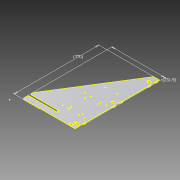
# Autodesk Inventor part: side_frame_v2
Saved by Autodesk Inventor 2013 (Build 170138000, 138)
## iProperties
Created: 2013-11-17
Part Number: side_frame_v2
Material: Generic
Document SubType Name: Modeling
Designer: Masta
Density: 1 g/cm^3
Author: Masta
Autodesk Inventor part; units mm, degrees
ref_plane "YZ Plane" through (0, 0, 0) normal (1, 0, 0) x (0, 1, 0)
ref_plane "XZ Plane" through (0, 0, 0) normal (0, 1, 0) x (-1, 0, 0)
ref_plane "XY Plane" through (0, 0, 0) normal (0, 0, 1) x (1, 0, 0)
sketch "Sketch1" plane through (0, 0, 0) normal (0, 0, 1) x (1, 0, 0)
  line L0 (255.7808, 350.0828) -> (255.7808, 358.8828)
  line L1 (251.6808, 67.29) -> (255.7808, 67.29)
  line L2 (255.7808, 67.29) -> (255.7808, 76.09)
  line L3 (255.7808, 76.09) -> (251.6808, 76.09)
  line L4 (251.6808, 76.09) -> (251.6808, 194.9901)
  line L5 (251.6808, 32.5401) -> (100.8808, 32.5401)
  line L6 (231.7439, 44.5401) -> (223.7479, 44.5401)
  line L7 (230.5808, 213.3401) -> (234.5808, 213.3401)
  line L8 (234.5808, 211.5401) -> (239.6808, 211.5401)
  line L9 (251.6808, 57.7345) -> (239.6808, 57.7345)
  line L10 (239.6808, 57.7345) -> (239.6808, 59.5345)
  line L11 (230.5808, 53.3345) -> (234.5808, 53.3345)
  line L12 (234.5808, 51.5345) -> (239.6808, 51.5345)
  line L13 (239.6808, 59.5345) -> (234.5808, 59.5345)
  line L14 (234.5808, 53.3345) -> (234.5808, 51.5345)
  line L15 (239.6808, 53.3345) -> (251.6808, 53.3345)
  line L16 (239.6808, 51.5345) -> (239.6808, 53.3345)
  line L17 (251.6808, 57.7345) -> (251.6808, 67.29)
  line L18 (251.6808, 217.7401) -> (239.6808, 217.7401)
  line L19 (255.7808, 236.0901) -> (251.6808, 236.0901)
  line L20 (251.6808, 236.0901) -> (251.6808, 350.0828)
  line L21 (255.7808, 203.7901) -> (251.6808, 203.7901)
  line L22 (251.6808, 194.9901) -> (255.7808, 194.9901)
  line L23 (255.7808, 194.9901) -> (255.7808, 203.7901)
  line L24 (251.6808, 227.2901) -> (251.6808, 217.7401)
  line L25 (251.6808, 213.3401) -> (251.6808, 203.7901)
  line L26 (251.6808, 382.3828) -> (255.7808, 382.3828)
  line L27 (255.7808, 382.3828) -> (255.7808, 391.1828)
  line L28 (255.7808, 391.1828) -> (251.6808, 391.1828)
  line L29 (251.6808, 391.1828) -> (251.6808, 400.5401)
  line L30 (255.7808, 358.8828) -> (251.6808, 358.8828)
  line L31 (251.6808, 350.0828) -> (255.7808, 350.0828)
  line L32 (73.8808, 35.5401) -> (73.8808, 51.1401)
  line L33 (239.6808, 211.5401) -> (239.6808, 213.3401)
  line L34 (230.5808, 217.7401) -> (230.5808, 213.3401)
  line L35 (73.8808, 77.5401) -> (226.2808, 400.5401)
  line L36 (234.5808, 217.7401) -> (230.5808, 217.7401)
  line L37 (234.5808, 217.7401) -> (234.5808, 219.5401)
  line L38 (251.6808, 400.5401) -> (226.2808, 400.5401)
  line L39 (239.6808, 213.3401) -> (251.6808, 213.3401)
  line L40 (231.7439, 36.5395) -> (223.7482, 36.5395)
  line L41 (239.6808, 219.5401) -> (234.5808, 219.5401)
  line L42 (98.8808, 30.5401) -> (78.8808, 30.5401)
  line L43 (234.5808, 213.3401) -> (234.5808, 211.5401)
  line L44 (230.5808, 372.825) -> (230.5808, 368.425)
  line L45 (234.5808, 372.825) -> (230.5808, 372.825)
  line L46 (234.5808, 372.825) -> (234.5808, 374.625)
  line L47 (251.6808, 372.825) -> (239.6808, 372.825)
  line L48 (230.5808, 368.425) -> (234.5808, 368.425)
  line L49 (239.6808, 368.425) -> (251.6808, 368.425)
  line L50 (234.5808, 366.625) -> (239.6808, 366.625)
  line L51 (239.6808, 374.625) -> (234.5808, 374.625)
  line L52 (234.5808, 368.425) -> (234.5808, 366.625)
  line L53 (251.6808, 372.825) -> (251.6808, 382.3828)
  line L54 (251.6808, 368.425) -> (251.6808, 358.8828)
  line L55 (230.5808, 57.7345) -> (230.5808, 53.3345)
  line L56 (234.5808, 57.7345) -> (230.5808, 57.7345)
  line L57 (234.5808, 57.7345) -> (234.5808, 59.5345)
  line L58 (239.6808, 366.625) -> (239.6808, 368.425)
  line L59 (239.6808, 372.825) -> (239.6808, 374.625)
  line L60 (78.8808, 56.1401) -> (148.8808, 56.1401)
  line L61 (78.8808, 56.1401) -> (73.8808, 51.1401)
  line L62 (78.8808, 64.9401) -> (148.8808, 64.9401)
  line L63 (73.8808, 69.9401) -> (73.8808, 77.5401)
  line L64 (78.8808, 64.9401) -> (73.8808, 69.9401)
  line L65 (251.6808, 227.2901) -> (255.7808, 227.2901)
  line L66 (255.7808, 227.2901) -> (255.7808, 236.0901)
  line L67 (239.6808, 217.7401) -> (239.6808, 219.5401)
  line L68 (78.8808, 30.5401) -> (73.8808, 35.5401)
  line L69 (100.8808, 32.5401) -> (98.8808, 30.5401)
  line L70 (251.6808, 32.5401) -> (251.6808, 53.3345)
  line L71 (136.6808, 189.5401) -> (231.6808, 189.5401) construction
  line L72 (231.6808, 189.5401) -> (231.6808, 93.5401) construction
  line L73 (231.6808, 93.5401) -> (136.6808, 93.5401) construction
  line L74 (136.6808, 93.5401) -> (136.6808, 189.5401) construction
  line L75 (164.6808, 93.5401) -> (208.6808, 93.5401) construction
  line L76 (208.6808, 93.5401) -> (208.6808, 187.5401) construction
  line L77 (208.6808, 187.5401) -> (164.6808, 187.5401) construction
  line L78 (164.6808, 187.5401) -> (164.6808, 93.5401) construction
  line L79 (160.3808, 93.5401) -> (208.6808, 93.5401) construction
  line L80 (208.6808, 93.5401) -> (208.6808, 168.5401) construction
  line L81 (208.6808, 168.5401) -> (160.3808, 168.5401) construction
  line L82 (160.3808, 168.5401) -> (160.3808, 93.5401) construction
  line L83 (208.6808, 168.5401) -> (208.6808, 174.8401) construction
  arc A0 (148.8808, 56.1401) -> (148.8808, 64.9401) centre (148.8808, 60.5401) ccw
  arc A1 (231.7439, 36.5395) -> (231.7439, 44.5401) centre (231.7439, 40.5398) ccw
  arc A2 (223.7479, 44.5401) -> (223.7482, 36.5395) centre (223.7482, 40.5398) ccw
  point P0 (0, 0)
  point P1 (219.7479, 40.5401)
  dimension "d0" = 177.8
  dimension "d9" = 95
  dimension "d10" = 96
  dimension "d11" = 44
  dimension "d12" = 94
  dimension "d15" = 48.3
  dimension "d16" = 75
  dimension "d18" = 6.3
  dimension "d19" = 23
  dimension "d20" = 20
  dimension "d21" = 63
  dimension "d22" = 4.1
  dimension "d23" = 8.8
  constraints: 168 end point, 17 collinear, 11 coincident, 7 parallel, 7 point on circle, 5 tangent, 4 horizontal, 3 centre point, 3 perpendicular, 1 vertical
  measures "d0" distance between parallel lines of L32 L70
  measures "d9" distance of L72.end L73.end
  measures "d10" distance of L71.end L72.end
  measures "d11" distance of L77.end L76.end
  measures "d12" distance of L75.end L76.end
  measures "d15" distance of L81.end L80.end
  measures "d16" distance of L80.end L75.end
  measures "d18" distance of L80.end L83.end
  measures "d19" distance between parallel lines of L72 L80
  measures "d20" distance between parallel lines of L4 L72
  measures "d21" distance between parallel lines of L42 L73
  measures "d22" distance between parallel lines of L2 L17
  measures "d23" distance of L1.end L2.end
extrude "Extrusion1" add sketch "Sketch1" against normal blind 4
hole "Hole1" at (136.6808, 189.5401, 0) at (136.6808, 93.5401, 0) at (231.6808, 93.5401, 0) at (231.6808, 189.5401, 0) at (160.3808, 93.5401, 0) at (208.6808, 93.5401, 0) at (208.6808, 174.8401, 0) at (160.3808, 168.5401, 0) at (164.6808, 93.5401, 0) at (164.6808, 187.5401, 0) at (208.6808, 187.5401, 0) direction (0, 0, -1) diameter 3.6 end through all
sketch "Sketch2" plane through (0, 0, 0) normal (0, 0, 1) x (1, 0, 0)
  line L0 (78.8808, 64.9401) -> (148.8808, 64.9401) projected
  line L1 (251.6808, 76.09) -> (251.6808, 194.9901) projected
  line L2 (162.1808, 104.9401) -> (212.1808, 104.9401) construction
  line L3 (212.1808, 104.9401) -> (212.1808, 254.9401) construction
  line L4 (212.1808, 254.9401) -> (162.1808, 254.9401) construction
  line L5 (162.1808, 254.9401) -> (162.1808, 104.9401) construction
  line L6 (162.1808, 104.9401) -> (212.1808, 254.9401) construction
  line L7 (212.1808, 104.9401) -> (162.1808, 254.9401) construction
  line L8 (129.6808, 69.9401) -> (244.6808, 69.9401) construction
  line L9 (244.6808, 69.9401) -> (244.6808, 289.9401) construction
  line L10 (244.6808, 289.9401) -> (129.6808, 289.9401) construction
  line L11 (129.6808, 289.9401) -> (129.6808, 69.9401) construction
  line L12 (129.6808, 69.9401) -> (244.6808, 289.9401) construction
  line L13 (244.6808, 69.9401) -> (129.6808, 289.9401) construction
  point P0 (0, 0)
  point P1 (187.1808, 179.9401)
  point P2 (187.1808, 179.9401)
  dimension "d33" = 50
  dimension "d34" = 150
  dimension "d35" = 115
  dimension "d36" = 220
  dimension "d37" = 5
  dimension "d38" = 7
  constraints: 24 end point, 5 midpoint, 4 coincident, 4 parallel, 2 horizontal, 2 perpendicular
  measures "d33" distance of L4.end L3.end
  measures "d34" distance of L3.end L2.end
  measures "d35" distance of L10.end L9.end
  measures "d36" distance of L9.end L8.end
  measures "d37" distance between parallel lines of L8 L0
  measures "d38" distance between parallel lines of L1 L9
hole "Hole2" at (162.1808, 254.9401, 0) at (162.1808, 104.9401, 0) at (212.1808, 104.9401, 0) at (212.1808, 254.9401, 0) direction (0, 0, -1) diameter 4.6 end through all
sketch "Sketch3" plane through (0, 0, 0) normal (0, 0, 1) x (1, 0, 0)
  line L0 (226.2808, 400.5401) -> (73.8808, 77.5401) projected
  line L1 (73.8808, 77.5401) -> (73.8808, 69.9401) projected
  line L2 (73.8808, 69.9401) -> (78.8808, 64.9401) projected
  line L3 (78.8808, 56.1401) -> (73.8808, 51.1401) projected
  line L4 (73.8808, 51.1401) -> (73.8808, 35.5401) projected
  line L5 (73.8808, 35.5401) -> (78.8808, 30.5401) projected
  line L6 (98.8808, 30.5401) -> (100.8808, 32.5401) projected
  line L7 (234.5808, 374.625) -> (239.6808, 374.625) projected
  line L8 (78.8808, 64.9401) -> (28.8808, 64.9401)
  line L9 (28.8808, 64.9401) -> (23.8808, 69.9401)
  line L10 (23.8808, 77.5401) -> (23.8808, 69.9401)
  line L11 (23.8808, 77.5401) -> (226.2808, 400.5401)
  line L12 (78.8808, 56.1401) -> (28.8808, 56.1401)
  line L13 (28.8808, 56.1401) -> (23.8808, 51.1401)
  line L14 (23.8808, 51.1401) -> (23.8808, 35.5401)
  line L15 (78.8808, 30.5401) -> (28.8808, 30.5401)
  line L16 (23.8808, 35.5401) -> (28.8808, 30.5401)
  point P0 (0, 0)
  point P1 (230.5808, 53.3345)
  point P2 (234.5808, 51.5345)
  point P3 (239.6808, 51.5345)
  point P4 (239.6808, 59.5345)
  point P5 (234.5808, 59.5345)
  point P6 (230.5808, 57.7345)
  point P7 (251.6808, 67.29)
  point P8 (251.6808, 76.09)
  point P9 (251.6808, 194.9901)
  point P10 (251.6808, 203.7901)
  point P11 (239.6808, 211.5401)
  point P12 (234.5808, 211.5401)
  point P13 (230.5808, 213.3401)
  point P14 (230.5808, 217.7401)
  point P15 (234.5808, 219.5401)
  point P16 (239.6808, 219.5401)
  point P17 (251.6808, 227.2901)
  point P18 (251.6808, 236.0901)
  point P19 (251.6808, 350.0828)
  point P20 (251.6808, 358.8828)
  point P21 (251.6808, 382.3828)
  point P22 (251.6808, 391.1828)
  point P23 (230.5808, 372.825)
  point P24 (230.5808, 368.425)
  point P25 (234.5808, 366.625)
  point P26 (239.6808, 366.625)
  dimension "d46" = 50
  dimension "d47" = 5
  dimension "d48" = 7.6
  constraints: 18 end point, 7 perpendicular, 2 coincident, 1 parallel
  measures "d46" distance of L2.end L8.end
  measures "d47" horizontal distance of L8.end L9.end
  measures "d48" distance of L10.start L9.end
extrude "Extrusion2" add sketch "Sketch3" against normal up to surface (4 mm away)
hole "Hole3" at (230.5808, 53.3345, 0) at (234.5808, 51.5345, 0) at (239.6808, 51.5345, 0) at (239.6808, 59.5345, 0) at (234.5808, 59.5345, 0) at (230.5808, 57.7345, 0) at (251.6808, 67.29, 0) at (251.6808, 76.09, 0) at (251.6808, 194.9901, 0) at (251.6808, 203.7901, 0) at (239.6808, 211.5401, 0) at (234.5808, 211.5401, 0) at (230.5808, 213.3401, 0) at (230.5808, 217.7401, 0) at (234.5808, 219.5401, 0) at (239.6808, 219.5401, 0) at (251.6808, 227.2901, 0) at (251.6808, 236.0901, 0) at (251.6808, 350.0828, 0) at (251.6808, 358.8828, 0) at (251.6808, 382.3828, 0) at (251.6808, 391.1828, 0) at (239.6808, 374.625, 0) at (234.5808, 374.625, 0) at (230.5808, 372.825, 0) at (230.5808, 368.425, 0) at (234.5808, 366.625, 0) at (239.6808, 366.625, 0) direction (0, 0, -1) diameter 1 end through all
sketch "Sketch4" plane through (0, 0, 0) normal (0, 0, 1) x (1, 0, 0)
  arc A0 (234.5808, 367.125) -> (235.0808, 366.625) centre (234.5808, 366.625) ccw projected
  line L0 (234.5808, 367.125) -> (234.5808, 368.425) projected
  line L1 (234.5808, 368.425) -> (231.0808, 368.425) projected
  arc A1 (230.5808, 368.925) -> (231.0808, 368.425) centre (230.5808, 368.425) ccw projected
  line L2 (230.5808, 368.925) -> (230.5808, 372.325) projected
  arc A2 (231.0808, 372.825) -> (230.5808, 372.325) centre (230.5808, 372.825) ccw projected
  line L3 (231.0808, 372.825) -> (234.5808, 372.825) projected
  line L4 (234.5808, 372.825) -> (234.5808, 374.125) projected
  arc A3 (235.0808, 374.625) -> (234.5808, 374.125) centre (234.5808, 374.625) ccw projected
  line L5 (235.0808, 374.625) -> (239.1808, 374.625) projected
  arc A4 (239.6808, 374.125) -> (239.1808, 374.625) centre (239.6808, 374.625) ccw projected
  line L6 (239.6808, 374.125) -> (239.6808, 372.825) projected
  line L7 (239.6808, 372.825) -> (251.6808, 372.825) projected
  line L8 (251.6808, 372.825) -> (251.6808, 381.8828) projected
  arc A5 (252.1808, 382.3828) -> (251.6808, 381.8828) centre (251.6808, 382.3828) ccw projected
  line L9 (252.1808, 382.3828) -> (255.7808, 382.3828) projected
  line L10 (255.7808, 382.3828) -> (255.7808, 391.1828) projected
  line L11 (255.7808, 391.1828) -> (252.1808, 391.1828) projected
  arc A6 (251.6808, 391.6828) -> (252.1808, 391.1828) centre (251.6808, 391.1828) ccw projected
  line L12 (251.6808, 391.6828) -> (251.6808, 400.5401) projected
  line L13 (251.6808, 400.5401) -> (226.2808, 400.5401) projected
  line L14 (226.2808, 400.5401) -> (23.8808, 77.5401) projected
  line L15 (23.8808, 77.5401) -> (23.8808, 69.9401) projected
  line L16 (23.8808, 69.9401) -> (28.8808, 64.9401) projected
  line L17 (28.8808, 64.9401) -> (148.8808, 64.9401) projected
  arc A7 (148.8808, 56.1401) -> (148.8808, 64.9401) centre (148.8808, 60.5401) ccw projected
  line L18 (148.8808, 56.1401) -> (28.8808, 56.1401) projected
  line L19 (28.8808, 56.1401) -> (23.8808, 51.1401) projected
  line L20 (23.8808, 51.1401) -> (23.8808, 35.5401) projected
  line L21 (23.8808, 35.5401) -> (28.8808, 30.5401) projected
  line L22 (28.8808, 30.5401) -> (98.8808, 30.5401) projected
  line L23 (98.8808, 30.5401) -> (100.8808, 32.5401) projected
  line L24 (100.8808, 32.5401) -> (251.6808, 32.5401) projected
  line L25 (251.6808, 32.5401) -> (251.6808, 53.3345) projected
  line L26 (251.6808, 53.3345) -> (239.6808, 53.3345) projected
  line L27 (239.6808, 53.3345) -> (239.6808, 52.0345) projected
  arc A8 (239.1808, 51.5345) -> (239.6808, 52.0345) centre (239.6808, 51.5345) ccw projected
  line L28 (239.1808, 51.5345) -> (235.0808, 51.5345) projected
  arc A9 (234.5808, 52.0345) -> (235.0808, 51.5345) centre (234.5808, 51.5345) ccw projected
  line L29 (234.5808, 52.0345) -> (234.5808, 53.3345) projected
  line L30 (234.5808, 53.3345) -> (231.0808, 53.3345) projected
  arc A10 (230.5808, 53.8345) -> (231.0808, 53.3345) centre (230.5808, 53.3345) ccw projected
  line L31 (230.5808, 53.8345) -> (230.5808, 57.2345) projected
  arc A11 (231.0808, 57.7345) -> (230.5808, 57.2345) centre (230.5808, 57.7345) ccw projected
  line L32 (231.0808, 57.7345) -> (234.5808, 57.7345) projected
  line L33 (234.5808, 57.7345) -> (234.5808, 59.0345) projected
  arc A12 (235.0808, 59.5345) -> (234.5808, 59.0345) centre (234.5808, 59.5345) ccw projected
  line L34 (235.0808, 59.5345) -> (239.1808, 59.5345) projected
  arc A13 (239.6808, 59.0345) -> (239.1808, 59.5345) centre (239.6808, 59.5345) ccw projected
  line L35 (239.6808, 59.0345) -> (239.6808, 57.7345) projected
  line L36 (239.6808, 57.7345) -> (251.6808, 57.7345) projected
  line L37 (251.6808, 57.7345) -> (251.6808, 66.79) projected
  arc A14 (252.1808, 67.29) -> (251.6808, 66.79) centre (251.6808, 67.29) ccw projected
  line L38 (252.1808, 67.29) -> (255.7808, 67.29) projected
  line L39 (255.7808, 67.29) -> (255.7808, 76.09) projected
  line L40 (255.7808, 76.09) -> (252.1808, 76.09) projected
  arc A15 (251.6808, 76.59) -> (252.1808, 76.09) centre (251.6808, 76.09) ccw projected
  line L41 (251.6808, 76.59) -> (251.6808, 194.4901) projected
  arc A16 (252.1808, 194.9901) -> (251.6808, 194.4901) centre (251.6808, 194.9901) ccw projected
  line L42 (252.1808, 194.9901) -> (255.7808, 194.9901) projected
  line L43 (255.7808, 194.9901) -> (255.7808, 203.7901) projected
  line L44 (255.7808, 203.7901) -> (252.1808, 203.7901) projected
  arc A17 (251.6808, 204.2901) -> (252.1808, 203.7901) centre (251.6808, 203.7901) ccw projected
  line L45 (251.6808, 204.2901) -> (251.6808, 213.3401) projected
  line L46 (251.6808, 213.3401) -> (239.6808, 213.3401) projected
  line L47 (239.6808, 213.3401) -> (239.6808, 212.0401) projected
  arc A18 (239.1808, 211.5401) -> (239.6808, 212.0401) centre (239.6808, 211.5401) ccw projected
  line L48 (239.1808, 211.5401) -> (235.0808, 211.5401) projected
  arc A19 (234.5808, 212.0401) -> (235.0808, 211.5401) centre (234.5808, 211.5401) ccw projected
  line L49 (234.5808, 212.0401) -> (234.5808, 213.3401) projected
  line L50 (234.5808, 213.3401) -> (231.0808, 213.3401) projected
  arc A20 (230.5808, 213.8401) -> (231.0808, 213.3401) centre (230.5808, 213.3401) ccw projected
  line L51 (230.5808, 213.8401) -> (230.5808, 217.2401) projected
  arc A21 (231.0808, 217.7401) -> (230.5808, 217.2401) centre (230.5808, 217.7401) ccw projected
  line L52 (231.0808, 217.7401) -> (234.5808, 217.7401) projected
  line L53 (234.5808, 217.7401) -> (234.5808, 219.0401) projected
  arc A22 (235.0808, 219.5401) -> (234.5808, 219.0401) centre (234.5808, 219.5401) ccw projected
  line L54 (235.0808, 219.5401) -> (239.1808, 219.5401) projected
  arc A23 (239.6808, 219.0401) -> (239.1808, 219.5401) centre (239.6808, 219.5401) ccw projected
  line L55 (239.6808, 219.0401) -> (239.6808, 217.7401) projected
  line L56 (239.6808, 217.7401) -> (251.6808, 217.7401) projected
  line L57 (251.6808, 217.7401) -> (251.6808, 226.7901) projected
  arc A24 (252.1808, 227.2901) -> (251.6808, 226.7901) centre (251.6808, 227.2901) ccw projected
  line L58 (252.1808, 227.2901) -> (255.7808, 227.2901) projected
  line L59 (255.7808, 227.2901) -> (255.7808, 236.0901) projected
  line L60 (255.7808, 236.0901) -> (252.1808, 236.0901) projected
  arc A25 (251.6808, 236.5901) -> (252.1808, 236.0901) centre (251.6808, 236.0901) ccw projected
  line L61 (251.6808, 236.5901) -> (251.6808, 349.5828) projected
  arc A26 (252.1808, 350.0828) -> (251.6808, 349.5828) centre (251.6808, 350.0828) ccw projected
  line L62 (252.1808, 350.0828) -> (255.7808, 350.0828) projected
  line L63 (255.7808, 350.0828) -> (255.7808, 358.8828) projected
  line L64 (255.7808, 358.8828) -> (252.1808, 358.8828) projected
  arc A27 (251.6808, 359.3828) -> (252.1808, 358.8828) centre (251.6808, 358.8828) ccw projected
  line L65 (251.6808, 359.3828) -> (251.6808, 368.425) projected
  line L66 (251.6808, 368.425) -> (239.6808, 368.425) projected
  line L67 (239.6808, 368.425) -> (239.6808, 367.125) projected
  arc A28 (239.1808, 366.625) -> (239.6808, 367.125) centre (239.6808, 366.625) ccw projected
  line L68 (239.1808, 366.625) -> (235.0808, 366.625) projected
  arc A29 (223.7479, 44.5401) -> (223.7482, 36.5395) centre (223.7482, 40.5398) ccw projected
  line L69 (223.7479, 44.5401) -> (231.7439, 44.5401) projected
  arc A30 (231.7439, 36.5395) -> (231.7439, 44.5401) centre (231.7439, 40.5398) ccw projected
  line L70 (231.7439, 36.5395) -> (223.7482, 36.5395) projected
  circle A31 centre (208.6808, 187.5401) radius 1.8 projected
  circle A32 centre (164.6808, 93.5401) radius 1.8 projected
  circle A33 centre (208.6808, 174.8401) radius 1.8 projected
  circle A34 centre (160.3808, 93.5401) radius 1.8 projected
  circle A35 centre (231.6808, 93.5401) radius 1.8 projected
  circle A36 centre (136.6808, 189.5401) radius 1.8 projected
  circle A37 centre (136.6808, 93.5401) radius 1.8 projected
  circle A38 centre (231.6808, 189.5401) radius 1.8 projected
  circle A39 centre (208.6808, 93.5401) radius 1.8 projected
  circle A40 centre (160.3808, 168.5401) radius 1.8 projected
  circle A41 centre (164.6808, 187.5401) radius 1.8 projected
  circle A42 centre (212.1808, 254.9401) radius 2.3 projected
  circle A43 centre (162.1808, 104.9401) radius 2.3 projected
  circle A44 centre (162.1808, 254.9401) radius 2.3 projected
  circle A45 centre (212.1808, 104.9401) radius 2.3 projected
  point P0 (0, 0)
  dimension "d58" = 370
  dimension "d59" = 231.9
  measures "d58" distance between parallel lines of L13 L22
  measures "d59" distance between parallel lines of L39 L20
body "Solid1"
